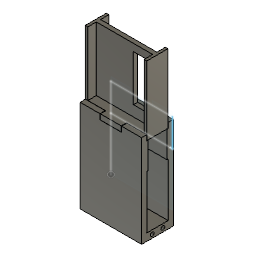
arduino_project_design (Autodesk Fusion 360 design; units mm, degrees)
Autodesk Fusion 360 part; units mm, degrees
sketch "Sketch3" plane through (0, 0, 0) normal (0, 0, 1) x (1, 0, 0)
  line L0 (29, 15) -> (-29, 15)
  line L1 (-29, 15) -> (-29, -15)
  line L2 (-29, -15) -> (29, -15)
  line L3 (29, -15) -> (29, 15)
  line L4 (29, 15) -> (-29, -15) construction
  line L5 (-29, 15) -> (29, -15) construction
  line L6 (10, 4) -> (-10, 4)
  line L7 (-10, 4) -> (-10, -4)
  line L8 (-10, -4) -> (10, -4)
  line L9 (10, -4) -> (10, 4)
  line L10 (10, 4) -> (-10, -4) construction
  line L11 (-10, 4) -> (10, -4) construction
  dimension "d5" = 58
  dimension "d6" = 30
  dimension "d7" = 20
  dimension "d8" = 8
  constraint horizontal L0
  constraint perpendicular L0 L1
  constraint parallel L0 L2
  constraint parallel L1 L3
  constraint coincident L4 origin
  constraint coincident L5 origin
  constraint horizontal L6
  constraint perpendicular L6 L7
  constraint parallel L6 L8
  constraint parallel L7 L9
  constraint coincident L10 origin
  constraint coincident L11 origin
  measures "d5" distance of L1.end L2.end
  measures "d6" distance of L0.end L1.end
  measures "d7" distance of L7.end L8.end
  measures "d8" distance of L6.end L7.end
extrude "Extrude1" add sketch "Sketch3" along normal blind 7 makes body 1
sketch "Sketch4" plane through (-29, 0, 0) normal (-1, 0, 0) x (0, -1, 0)
  line L0 (-15, 0) -> (15, 0)
  line L1 (15, 0) -> (15, 7)
  line L2 (15, 7) -> (-15, 7)
  line L3 (-15, 7) -> (-15, 0)
  line L4 (-15, 3.5) -> (-5, 3.5)
  line L5 (15, 3.5) -> (5, 3.5)
  circle A0 centre (-5, 3.5) radius 1.75
  circle A1 centre (5, 3.5) radius 1.75
  dimension "d11" = 10
  dimension "d12" = 10
  dimension "d13" = 3.5
  dimension "d14" = 3.5
  constraint midpoint L3 L4.start
  constraint perpendicular L1 L4
  constraint midpoint L1 L5.start
  constraint perpendicular L1 L5
  constraint coincident L4.end A0.centre
  constraint coincident L5.end A1.centre
  measures "d11" distance of L4.start L4.end
  measures "d12" distance of L5.start L5.end
  measures "d13" diameter of A0
extrude "Extrude2" cut sketch "Sketch4" against normal blind 58 contours A0 | A1 bodies 1
sketch "Sketch5" plane through (0, 0, 7) normal (0, 0, 1) x (-1, 0, 0)
  line L0 (-10, -4) -> (-10, 4)
  line L1 (-10, 4) -> (10, 4)
  line L2 (10, 4) -> (10, -4)
  line L3 (10, -4) -> (-10, -4)
  line L4 (-29, 15) -> (-29, -15)
  line L5 (-29, -15) -> (29, -15)
  line L6 (29, -15) -> (29, 15)
  line L7 (29, 15) -> (-29, 15)
  line L8 (-29, -15) -> (29, -15)
  line L9 (29, -15) -> (29, -10)
  line L10 (29, -10) -> (-29, -10)
  line L11 (-29, -10) -> (-29, -15)
  line L12 (-29, 15) -> (29, 15)
  line L13 (29, 15) -> (29, 10)
  line L14 (29, 10) -> (-29, 10)
  line L15 (-29, 10) -> (-29, 15)
  dimension "d17" = 5
  dimension "d18" = 5
  constraint horizontal L8
  constraint vertical L9
  constraint horizontal L10
  constraint vertical L11
  constraint coincident L4.end L5.start
  constraint horizontal L12
  constraint vertical L13
  constraint horizontal L14
  constraint vertical L15
  constraint coincident L4.start L7.end
  measures "d17" distance of L4.end L10.end
  measures "d18" distance of L4.start L14.end
extrude "Extrude3" add sketch "Sketch5" along normal blind 80 contours L4 L6 L7 L12 L13 L14 L15 | L4 L5 L6 L8 L9 L10 L11 bodies 1
sketch "Sketch6" plane through (0, 0, 87) normal (0, 0, 1) x (-1, 0, 0)
  line L0 (-29, 10) -> (29, 10)
  line L1 (29, 10) -> (29, 15)
  line L2 (29, 15) -> (-29, 15)
  line L3 (-29, 15) -> (-29, 10)
  line L4 (10, -15) -> (-10, -15)
  line L5 (-10, -15) -> (-10, -10)
  line L6 (-10, -10) -> (10, -10)
  line L7 (10, -10) -> (10, -15)
  line L8 (10, 10) -> (-10, 10)
  line L9 (-10, 10) -> (-10, 15)
  line L10 (-10, 15) -> (10, 15)
  line L11 (10, 15) -> (10, 10)
  constraint horizontal L4
  constraint vertical L5
  constraint horizontal L6
  constraint vertical L7
  constraint horizontal L8
  constraint vertical L9
  constraint horizontal L10
  constraint vertical L11
  constraint coincident L2 L9.end
  constraint coincident L0 L8.start
sketch "Sketch7" plane through (0, 0, 87) normal (0, 0, 1) x (-1, 0, 0)
  line L0 (-29, -10) -> (-29, -15)
  line L1 (-29, -15) -> (29, -15)
  line L2 (29, -15) -> (29, -10)
  line L3 (29, -10) -> (-29, -10)
  line L4 (29, -15) -> (-29, -15)
  line L5 (-29, -15) -> (-29, 15)
  line L6 (-29, 15) -> (29, 15)
  line L7 (29, 15) -> (29, -15)
  constraint horizontal L4
  constraint vertical L5
  constraint horizontal L6
  constraint vertical L7
  constraint coincident L1.end L2.start
extrude "Extrude4" add sketch "Sketch7" along normal blind 5 separate body makes body 2
extrude "Extrude5" cut sketch "Sketch6" against normal blind 5 contours L0 L2 L8 L9 L10 L11 | L4 L5 L6 L7 bodies 2 1
sketch "Sketch9" plane through (0, 0, 92) normal (0, 0, 1) x (-1, 0, 0)
  line L0 (29, 15) -> (-29, 15)
  line L1 (-29, 15) -> (-29, -15)
  line L2 (-29, -15) -> (29, -15)
  line L3 (29, -15) -> (29, 15)
  line L4 (29, -15) -> (10, -15)
  line L5 (10, -15) -> (10, -10)
  line L6 (10, -10) -> (29, -10)
  line L7 (29, -10) -> (29, -15)
  line L8 (-10, -15) -> (-29, -15)
  line L9 (-29, -15) -> (-29, -10)
  line L10 (-29, -10) -> (-10, -10)
  line L11 (-10, -10) -> (-10, -15)
  line L12 (-29, 10) -> (-10, 10)
  line L13 (-10, 10) -> (-10, 15)
  line L14 (-10, 15) -> (-29, 15)
  line L15 (-29, 15) -> (-29, 10)
  line L16 (10, 10) -> (29, 10)
  line L17 (29, 10) -> (29, 15)
  line L18 (29, 15) -> (10, 15)
  line L19 (10, 15) -> (10, 10)
  constraint horizontal L4
  constraint vertical L5
  constraint horizontal L6
  constraint vertical L7
  constraint coincident L2.end L3.start
  constraint horizontal L8
  constraint vertical L9
  constraint horizontal L10
  constraint vertical L11
  constraint coincident L1 L9.end
  constraint coincident L2 L8.start
  constraint horizontal L12
  constraint vertical L13
  constraint horizontal L14
  constraint vertical L15
  constraint coincident L0 L13.end
  constraint coincident L1 L12.start
  constraint horizontal L16
  constraint vertical L17
  constraint horizontal L18
  constraint vertical L19
  constraint coincident L0.start L3.end
extrude "Extrude6" cut sketch "Sketch9" against normal blind 5 contours L0 L3 L16 L17 L18 L19 | L0 L1 L12 L13 L14 L15 | L2 L3 L4 L5 L6 L7 | L1 L2 L8 L9 L10 L11 bodies 2 1
sketch "Sketch10" plane through (0, 0, 92) normal (0, 0, 1) x (-1, 0, 0)
  line L0 (10, 10) -> (10, 15)
  line L1 (10, 15) -> (-10, 15)
  line L2 (-10, 15) -> (-10, 10)
  line L3 (-10, 10) -> (-29, 10)
  line L4 (-29, 10) -> (-29, -10)
  line L5 (-29, -10) -> (-10, -10)
  line L6 (-10, -10) -> (-10, -15)
  line L7 (-10, -15) -> (10, -15)
  line L8 (10, -15) -> (10, -10)
  line L9 (10, -10) -> (29, -10)
  line L10 (29, -10) -> (29, 10)
  line L11 (29, 10) -> (10, 10)
  line L12 (-29, 10) -> (-29, -10)
  line L13 (-29, 0) -> (29, 0)
  line L14 (29, 0) -> (29, 2)
  line L15 (29, 2) -> (-29, 2)
  line L16 (-29, 2) -> (-29, -2)
  line L17 (-29, -2) -> (29, -2)
  line L18 (29, -2) -> (29, 2)
  dimension "d27" = 2
  dimension "d28" = 4
  constraint coincident L3.end L4.start
  constraint coincident L4.end L5.start
  constraint midpoint L12 L13.start
  constraint midpoint L10 L13.end
  constraint perpendicular L13 L14
  constraint horizontal L15
  constraint vertical L16
  constraint horizontal L17
  constraint vertical L18
  measures "d27" distance of L13.end L14.end
  measures "d28" distance of L14.end L17.end
extrude "Extrude7" add sketch "Sketch10" along normal blind 60 contours L4 L10 L12 L13 L14 L15 L16 L18 | L4 L10 L12 L13 L16 L17 L18 bodies 2
sketch "Sketch11" plane through (0, 0, 92) normal (0, 0, 1) x (-1, 0, 0)
  line L0 (-29, 2) -> (29, 2)
  line L1 (29, 2) -> (29, 10)
  line L2 (29, 10) -> (10, 10)
  line L3 (10, 10) -> (10, 15)
  line L4 (10, 15) -> (-10, 15)
  line L5 (-10, 15) -> (-10, 10)
  line L6 (-10, 10) -> (-29, 10)
  line L7 (-29, 10) -> (-29, 2)
  line L8 (-29, 10) -> (-26.5, 10)
  line L9 (-26.5, 10) -> (-26.5, 2)
  line L10 (-26.5, 2) -> (-29, 2)
  line L11 (-29, 2) -> (-29, 10)
  line L12 (-29, -10) -> (-26.5, -10)
  line L13 (-26.5, -10) -> (-26.5, -2)
  line L14 (-26.5, -2) -> (-29, -2)
  line L15 (-29, -2) -> (-29, -10)
  line L16 (29, -10) -> (26.5, -10)
  line L17 (26.5, -10) -> (26.5, -2)
  line L18 (26.5, -2) -> (29, -2)
  line L19 (29, -2) -> (29, -10)
  line L20 (29, 2) -> (26.5, 2)
  line L21 (26.5, 2) -> (26.5, 10)
  line L22 (26.5, 10) -> (29, 10)
  line L23 (29, 10) -> (29, 2)
  dimension "d37" = 2.5
  dimension "d38" = 2.5
  dimension "d39" = 8
  dimension "d40" = 2.5
  dimension "d41" = 8
  dimension "d42" = 2.5
  constraint horizontal L8
  constraint vertical L9
  constraint horizontal L10
  constraint vertical L11
  constraint coincident L6.end L7.start
  constraint horizontal L12
  constraint vertical L13
  constraint horizontal L14
  constraint vertical L15
  constraint horizontal L16
  constraint vertical L17
  constraint horizontal L18
  constraint vertical L19
  constraint horizontal L20
  constraint vertical L21
  constraint horizontal L22
  constraint vertical L23
  constraint coincident L0.end L1.start
  measures "d37" distance of L6.end L8.end
  measures "d38" distance of L12.start L12.end
  measures "d39" distance of L12.start L14.end
  measures "d40" distance of L16.start L16.end
  measures "d41" distance of L16.start L18.end
  measures "d42" distance of L0.end L20.end
extrude "Extrude8" add sketch "Sketch11" along normal blind 60 contours L0 L6 L7 L8 L9 L10 L11 | L0 L1 L2 L20 L21 L22 L23 | L12 L13 L14 L15 | L16 L17 L18 L19 bodies 2
sketch "Sketch12" plane through (0, -2, 0) normal (0, -1, 0) x (1, 0, 0)
  line L0 (26.5, 92) -> (26.5, 152)
  line L1 (26.5, 152) -> (-26.5, 152)
  line L2 (-26.5, 152) -> (-26.5, 92)
  line L3 (-26.5, 92) -> (26.5, 92)
  line L4 (-20.1432, 145.0863) -> (-26.5, 145.0863)
  line L5 (-26.5, 145.0863) -> (-26.5, 99.6355)
  line L6 (-26.5, 99.6355) -> (-20.1432, 99.6355)
  line L7 (-20.1432, 99.6355) -> (-20.1432, 145.0863)
  line L8 (26.5, 145.2014) -> (20.1432, 145.2014)
  line L9 (20.1432, 145.2014) -> (20.1432, 99.7506)
  line L10 (20.1432, 99.7506) -> (26.5, 99.7506)
  line L11 (26.5, 99.7506) -> (26.5, 145.2014)
  constraint horizontal L4
  constraint vertical L5
  constraint horizontal L6
  constraint vertical L7
  constraint coincident L2 L5.end
  constraint horizontal L8
  constraint vertical L9
  constraint horizontal L10
  constraint vertical L11
  constraint coincident L0 L8.start
  constraint equal L4 L8
  constraint equal L7 L9
extrude "Extrude9" cut sketch "Sketch12" against normal blind 5 contours L0 L8 L9 L10 L11 bodies 2
sketch "Sketch13" plane through (0, 10, 0) normal (0, -1, 0) x (1, 0, 0)
  line L0 (10, 87) -> (10, 82)
  line L1 (10, 82) -> (-10, 82)
  line L2 (-10, 82) -> (-10, 87)
  line L3 (-10, 87) -> (-29, 87)
  line L4 (-29, 87) -> (-29, 7)
  line L5 (-29, 7) -> (29, 7)
  line L6 (29, 7) -> (29, 87)
  line L7 (29, 87) -> (10, 87)
  line L8 (-29, 7) -> (-29, 57)
  line L9 (-29, 57) -> (29, 57)
  line L10 (29, 57) -> (29, 83)
  line L11 (29, 83) -> (-29, 83)
  line L12 (-29, 83) -> (-29, 57)
  dimension "d47" = 50
  dimension "d48" = 26
  constraint coincident L4.end L5.start
  constraint perpendicular L5 L8
  constraint horizontal L9
  constraint vertical L10
  constraint horizontal L11
  constraint vertical L12
  measures "d47" distance of L4.end L8.end
  measures "d48" distance of L8.end L11.end
extrude "Extrude10" add sketch "Sketch13" along normal blind 1 contours L0 L1 L2 L4 L6 L9 L10 L11 L12 | L0 L1 L2 L11 bodies 1
extrude "Extrude11" add sketch "Sketch13" against normal blind 1 from surface at 20 contours L0 L1 L2 L4 L6 L9 L10 L11 L12 bodies 1
sketch "Sketch14" plane through (0, 10, 0) normal (0, -1, 0) x (1, 0, 0)
  line L0 (10, 87) -> (-10, 87)
  line L1 (-10, 87) -> (-10, 82)
  line L2 (-10, 82) -> (10, 82)
  line L3 (10, 82) -> (10, 87)
  constraint horizontal L0
  constraint vertical L1
  constraint horizontal L2
  constraint vertical L3
extrude "Extrude12" cut sketch "Sketch14" along normal blind 26 bodies 1
sketch "Sketch15" plane through (0, 2, 0) normal (0, 1, 0) x (-1, 0, 0)
  line L0 (26.5, 152) -> (-26.5, 152)
  line L1 (-26.5, 152) -> (-26.5, 145.2014)
  line L2 (-26.5, 145.2014) -> (-20.1432, 145.2014)
  line L3 (-20.1432, 145.2014) -> (-20.1432, 99.7506)
  line L4 (-20.1432, 99.7506) -> (-26.5, 99.7506)
  line L5 (-26.5, 99.7506) -> (-26.5, 92)
  line L6 (-26.5, 92) -> (26.5, 92)
  line L7 (26.5, 92) -> (26.5, 152)
  line L8 (-26.5, 145.2014) -> (-8.3, 145.2014)
  line L9 (-8.3, 145.2014) -> (-8.3, 102.0014)
  line L10 (-8.3, 102.0014) -> (-26.5, 102.0014)
  line L11 (-26.5, 102.0014) -> (-26.5, 145.2014)
  dimension "d56" = 18.2
  dimension "d57" = 43.2
  constraint horizontal L8
  constraint vertical L9
  constraint horizontal L10
  constraint vertical L11
  constraint coincident L1.end L2.start
  measures "d56" distance of L1.end L8.end
  measures "d57" distance of L1.end L10.end
extrude "Extrude13" cut sketch "Sketch15" against normal blind 15 contours L3 L8 L9 L10 bodies 2
move_body "Move1" bodies 2 to x (1, 0, 0) y (0, 1, 0) z (0, 0, 1) at (100, 0, -80)
copy_body "Body->Comp1" bodies 2 removing the originals makes body 3 in component "Component"
copy_body "Body->Comp2" bodies 1 removing the originals makes body 4 in component "Component'"
sketch "Sketch16" plane through (7.5234, 0, 0) normal (-1, 0, 0) x (0, -1, 0)
  line L0 (-8.4129, 78.0371) -> (-13.4129, 78.0371)
  line L1 (-13.4129, 78.0371) -> (-13.4129, 73.0371)
  line L2 (-13.4129, 73.0371) -> (-7.4129, 73.0372)
  line L3 (-7.4129, 73.0372) -> (-7.4129, 74.0371)
  line L4 (-7.4129, 74.0371) -> (-8.4129, 74.0371)
  line L5 (-8.4129, 74.0371) -> (-8.4129, 78.0371)
  line L6 (-8.4129, 75.3627) -> (-8.4129, 73.1246)
  line L7 (-8.4129, 74.0371) -> (-7.4129, 74.0371)
  line L8 (-7.4129, 74.0371) -> (-7.4129, 73.0372)
  line L9 (-7.4129, 73.0372) -> (-8.4129, 73.0372)
  line L10 (-8.4129, 73.0372) -> (-8.4129, 74.0371)
  constraint coincident L5 L6.start
  constraint perpendicular L2 L6
  constraint horizontal L7
  constraint vertical L8
  constraint horizontal L9
  constraint vertical L10
  constraint coincident L2.end L3.start
  constraint coincident L4.end L5.start
extrude "Extrude1'" cut sketch "Sketch16" along normal blind 43 and the other way blind 27 contours L2 L3 L4 L6 L7 L8 L9 L10 sketch seen with x (1, 0, 0) y (0, 1, 0) z (0, 0, 1) at (2.4766, 1.5871, 8.9629) bodies 4 in component "Component'"
sketch "Sketch17" plane through (7.5234, 0, 0) normal (-1, 0, 0) x (0, -1, 0)
  line L0 (16.5871, 78.0371) -> (11.5871, 78.0371)
  line L1 (11.5871, 78.0371) -> (11.5871, 74.0371)
  line L2 (11.5871, 74.0371) -> (10.5871, 74.0371)
  line L3 (10.5871, 74.0371) -> (10.5871, 73.0371)
  line L4 (10.5871, 73.0371) -> (16.5871, 73.0371)
  line L5 (16.5871, 73.0371) -> (16.5871, 78.0371)
  line L6 (11.5871, 75.433) -> (11.5871, 73.0371)
  line L7 (10.5871, 74.0371) -> (11.5871, 74.0371)
  line L8 (11.5871, 74.0371) -> (11.5871, 73.0371)
  line L9 (11.5871, 73.0371) -> (10.5871, 73.0371)
  line L10 (10.5871, 73.0371) -> (10.5871, 74.0371)
  constraint coincident L1 L6.start
  constraint coincident L4 L6.end
  constraint perpendicular L4 L6
  constraint horizontal L7
  constraint vertical L8
  constraint horizontal L9
  constraint vertical L10
  constraint coincident L2.end L3.start
extrude "Extrude2'" cut sketch "Sketch17" along normal blind 64 and the other way blind 28 contours L2 L3 L4 L6 L7 L8 L9 L10 sketch seen with x (1, 0, 0) y (0, 1, 0) z (0, 0, 1) at (2.4766, 1.5871, 8.9629) bodies 4 in component "Component'"
component "Component" placed x (1, 0, 0) y (0, 1, 0) z (0, 0, 1) at (0, 0, 0)
component "Component'" placed x (1, 0, 0) y (0, 1, 0) z (0, 0, 1) at (-2.4766, -1.5871, -8.9629)
